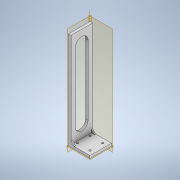
# Autodesk Inventor part: IDOM_infrared_fixture2
Saved by Autodesk Inventor 2022 (Build 260153000, 153)
## iProperties
Created: 2022-07-06
Part Number: IDOM_infrared_fixture2
Material: Generic
Document SubType Name: Modeling
Designer: dovalle
Density: 1 g/cm^3
Appearance: Default
Author: dovalle
Autodesk Inventor part; units mm, degrees
sketch "Sketch1" plane through (0, 0, 0) normal (0, 0, 1) x (1, 0, 0)
  line L0 (0, 0) -> (34, 0)
  line L1 (34, 0) -> (34, 4)
  line L2 (34, 4) -> (4, 4)
  line L3 (4, 4) -> (4, 154)
  line L4 (4, 154) -> (0, 154)
  line L5 (0, 154) -> (0, 0)
  dimension "d2" = 34
  dimension "d3" = 4
  dimension "d4" = 30
  dimension "d5" = 150
  dimension "d6" = 4
  constraints: 12 end point, 3 perpendicular, 1 horizontal, 1 vertical
  measures "d2" distance of L0.start L0.end
  measures "d3" distance of L0.end L1.end
  measures "d4" distance of L1.end L2.end
  measures "d5" distance of L2.end L3.end
  measures "d6" distance of L3.end L4.end
extrude "Extrusion1" add sketch "Sketch1" along normal blind 34
sketch "Sketch3" plane through (4, 4, 0) normal (1, 0, 0) x (0, 0, -1)
  line L0 (0, 0) -> (-34, 0) projected
  line L1 (0, 150) -> (-34, 150) projected
  arc A0 (-27, 20) -> (-7, 20) centre (-17, 20) ccw
  arc A1 (-7, 130) -> (-27, 130) centre (-17, 130) ccw
  line L2 (-27, 20) -> (-27, 130)
  line L3 (-7, 130) -> (-7, 20)
  point P0 (0, -4)
  constraints: 4 end point, 4 point on circle, 2 centre point, 2 vertical
extrude "Extrusion3" cut sketch "Sketch3" against normal blind 20
sketch "Sketch4" plane through (0, 0, 0) normal (0, -1, 0) x (1, 0, 0)
  line L0 (0, 0) -> (34, 0) projected
  line L1 (34, 0) -> (34, 34) projected
  line L2 (0, 34) -> (34, 34) projected
  line L3 (0, 0) -> (0, 34) projected
  line L4 (4, 34) -> (0, 34) projected
  line L5 (34, 0) -> (34, 34) projected
  circle A0 centre (26.9999, 26.9999) radius 1.5
  circle A1 centre (26.9999, 7.0001) radius 1.5
  circle A2 centre (7.0001, 26.9999) radius 1.5
  circle A3 centre (7.0001, 7.0001) radius 1.5
  dimension "d28" = 3
  dimension "d29" = 3
  dimension "d30" = 3
  dimension "d31" = 3
  constraints: 4 centre point
  measures "d28" diameter of A0
  measures "d29" diameter of A1
  measures "d30" diameter of A2
  measures "d31" diameter of A3
extrude "Extrusion4" cut sketch "Sketch4" against normal blind 10 contours A0 | A1 | A2 | A3
sketch "Sketch5" plane through (4, 4, 0) normal (0, 1, 0) x (1, 0, 0)
  line L0 (0, 0) -> (0, -34) projected
  line L1 (36.8, 0) -> (-10.8, 0) projected
  line L2 (30, 0) -> (0, 0) projected
  line L3 (0, 0) -> (0, -2)
  line L4 (0, 0) -> (0, -34) projected
  line L5 (0, -2) -> (5, -2)
  line L6 (5, -2) -> (5, 0)
  line L7 (30, -34) -> (0, -34) projected
  line L8 (0, -34) -> (0, -32)
  line L9 (0, -32) -> (5, -32)
  line L10 (5, -32) -> (5, -34)
  line L11 (5, -34) -> (0, -34)
  point P0 (-4, 0)
  dimension "d34" = 2
  dimension "d35" = 5
  dimension "d36" = 2
  dimension "d37" = 5
  constraints: 14 end point, 5 perpendicular, 3 point on line
  measures "d34" distance of L0.start L3.end
  measures "d35" distance of L3.end L5.end
  measures "d36" distance of L0.end L8.end
  measures "d37" distance of L8.end L9.end
extrude "Extrusion5" add sketch "Sketch5" along normal blind 5
sketch "Sketch6" plane through (0, 0, 0) normal (0, 0, -1) x (-1, 0, 0)
  line L0 (-34, 0) -> (-34, 4) projected
  line L1 (0, 0) -> (-34, 0) projected
  line L2 (0, 154) -> (0, 0) projected
  line L3 (-4, 154) -> (0, 154) projected
  line L4 (-4, 9) -> (-4, 154) projected
  line L5 (-9, 9) -> (-4, 9) projected
  line L6 (-9, 4) -> (-9, 9) projected
  line L7 (-34, 4) -> (-9, 4) projected
  line L8 (-4, 9) -> (-4, 4) projected
  line L9 (-9, 4) -> (-4, 9)
  line L10 (-4, 9) -> (-9, 9) projected
  line L11 (-4, 9) -> (-9, 9)
  line L12 (-9, 4) -> (-9, 9) projected
  line L13 (-9, 9) -> (-9, 4)
  constraints: 6 end point, 2 collinear
extrude "Extrusion6" cut sketch "Sketch6" against normal blind 4000 contours L6 L5 L9
body "Solid1"
